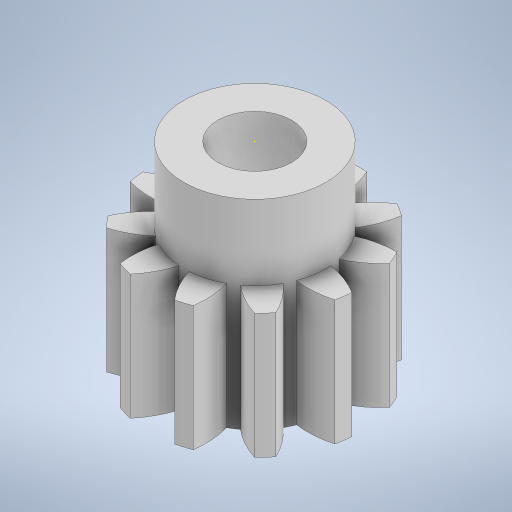
# Autodesk Inventor part: piniongear
Saved by Autodesk Inventor 2024 (Build 280153000, 153)
## iProperties
Created: 2024-05-02
Part Number: piniongear
Material: Generic
Document SubType Name: Modeling
Designer: maja6
Density: 1 g/cm^3
Appearance: Default
Author: maja6
Autodesk Inventor part; units mm, degrees
ref_plane "YZ Plane" through (0, 0, 0) normal (1, 0, 0) x (0, 1, 0)
ref_plane "XZ Plane" through (0, 0, 0) normal (0, 1, 0) x (-1, 0, 0)
ref_plane "XY Plane" through (0, 0, 0) normal (0, 0, 1) x (1, 0, 0)
sketch "Sketch1" plane through (0, 0, 0) normal (0, 0, 1) x (1, 0, 0)
  circle A0 centre (0, 0) radius 8.5
  dimension "d0" = 17
  constraints: 1 centre point, 1 coincident
  measures "d0" diameter of A0
extrude "Extrusion1" add sketch "Sketch1" along normal blind 5
spur gear teeth "Spur Gear1" teeth 11 pitch diameter 13.75 tip diameter 16.7792 root diameter 11.375 face width 5 trims to tip circle yes start plane through (0, 0, 5) normal (0, 0, 1) x (1, 0, 0)
sketch "Sketch2" plane through (0, 0, 5) normal (0, 0, 1) x (1, 0, 0)
  circle A0 centre (0, 0) radius 3.05
  circle A1 centre (0, 0) radius 5.6875
  point P0 (4.5531, 3.4084)
  dimension "d3" = 6.1
  constraints: 2 coincident, 1 centre point, 3 other
  measures "d3" diameter of A0
extrude "Extrusion2" add sketch "Sketch2" along normal blind 6
extrude "Extrusion3" cut sketch "Sketch2" against normal blind 6 contours A0
sketch "Sketch3" plane through (0, 0, 5) normal (0, 0, 1) x (1, 0, 0)
  line L0 (-1.9876, 4.927) -> (1.6861, 4.927)
  line L1 (1.6861, 4.927) -> (1.6861, 4.0217)
  line L2 (1.6861, 4.0217) -> (-1.9876, 4.0217)
  line L3 (-1.9876, 4.0217) -> (-1.9876, 4.927)
  point P0 (0, 0)
  constraints: 8 end point, 2 parallel, 1 horizontal, 1 perpendicular
sketch "Sketch4" plane through (0, 0, 11) normal (0, 0, 1) x (1, 0, 0)
  arc A0 (-1.209, 5.5575) -> (-1.9876, 5.3289) centre (0, 0) ccw projected
  line L0 (-1.9876, 5.3289) -> (1.9927, 5.3289)
  line L1 (1.9927, 5.3289) -> (1.9927, 4.1825)
  line L2 (1.9927, 4.1825) -> (-1.9876, 4.1825)
  line L3 (-1.9876, 4.1825) -> (-1.9876, 5.3289)
  constraints: 8 end point, 2 parallel, 1 horizontal, 1 perpendicular
extrude "Extrusion4" add sketch "Sketch4" along normal blind 6
sketch "Sketch5" plane through (-1.9876, 5.3289, 11) normal (0, 1, 0) x (1, 0, 0)
  circle A0 centre (1.9876, 3.0949) radius 1.5
  point P0 (1.9876, 11)
  dimension "d10" = 3
  constraints: 1 centre point
  measures "d10" diameter of A0
extrude "Extrusion5" cut sketch "Sketch5" along normal mid plane 30
sketch "Sketch6" plane through (-1.9876, 5.3289, 11) normal (0, 1, 0) x (1, 0, 0)
  line L0 (0, 0) -> (0, -6) projected
  line L1 (0, 0) -> (8.0095, 0)
  line L2 (8.0095, 0) -> (8.0095, -7.9416)
  line L3 (8.0095, -7.9416) -> (0, -7.9416)
  line L4 (0, -7.9416) -> (0, 0)
  point P0 (1.9876, 11)
  constraints: 8 end point, 2 parallel, 1 horizontal, 1 perpendicular
extrude "Extrusion6" cut sketch "Sketch6" against normal blind 30
thread "Thread1" size "M3x0.5" class "6H" standard "ANSI Metric M Profile" full length
thread "Thread2" size "M3x0.5" class "6H" standard "ANSI Metric M Profile" full length
sketch "Sketch7" plane through (0, 0, 11) normal (0, 0, 1) x (1, 0, 0)
  circle A0 centre (0, 0) radius 3.05
  circle A1 centre (0, 0) radius 2.95
  dimension "d19" = 5.9
  constraints: 2 centre point, 2 coincident
  measures "d19" diameter of A1
extrude "Extrusion7" add sketch "Sketch7" against normal blind 11
sketch "Sketch8" plane through (0, 0, 11) normal (0, 0, 1) x (1, 0, 0)
  circle A0 centre (0, 0) radius 2.95
  circle A1 centre (0, 0) radius 5.6875
  constraints: 2 centre point, 2 coincident
extrude "Extrusion8" add sketch "Sketch8" against normal blind 10
extrude "Extrusion9" add sketch "Sketch3" along normal blind 10
sketch "Sketch9" plane through (0, 0, 0) normal (0, 0, -1) x (-1, 0, 0)
  arc A0 (4.5531, 3.4084) -> (4.0217, 4.0217) centre (0, 0) ccw projected
  arc A1 (7.3634, 4.0207) -> (4.5531, 3.4084) centre (7.409, -2.9439) ccw projected
  arc A2 (7.8606, 2.9319) -> (7.3634, 4.0207) centre (0, 0) ccw projected
  arc A3 (5.5575, 1.209) -> (7.8606, 2.9319) centre (2.627, 7.5272) ccw projected
  arc A4 (5.673, 0.4057) -> (5.5575, 1.209) centre (0, 0) ccw projected
  arc A5 (8.3682, -0.5985) -> (5.673, 0.4057) centre (4.6413, -6.4821) ccw projected
  arc A6 (8.1979, -1.7833) -> (8.3682, -0.5985) centre (0, 0) ccw projected
  arc A7 (5.3289, -1.9876) -> (8.1979, -1.7833) centre (6.2795, 4.912) ccw projected
  arc A8 (4.9918, -2.7257) -> (5.3289, -1.9876) centre (0, 0) ccw projected
  arc A9 (6.7162, -5.0277) -> (4.9918, -2.7257) centre (0.4, -7.9624) ccw projected
  arc A10 (5.9324, -5.9324) -> (6.7162, -5.0277) centre (0, 0) ccw projected
  arc A11 (3.4084, -4.5531) -> (5.9324, -5.9324) centre (7.9383, 0.7373) ccw projected
  arc A12 (2.7257, -4.9918) -> (3.4084, -4.5531) centre (0, 0) ccw projected
  arc A13 (2.9319, -7.8606) -> (2.7257, -4.9918) centre (-3.9683, -6.9146) ccw projected
  arc A14 (1.7833, -8.1979) -> (2.9319, -7.8606) centre (0, 0) ccw projected
  arc A15 (0.4057, -5.673) -> (1.7833, -8.1979) centre (7.0767, -3.6715) ccw projected
  arc A16 (-0.4057, -5.673) -> (0.4057, -5.673) centre (0, 0) ccw projected
  arc A17 (-1.7833, -8.1979) -> (-0.4057, -5.673) centre (-7.0767, -3.6715) ccw projected
  arc A18 (-2.9319, -7.8606) -> (-1.7833, -8.1979) centre (0, 0) ccw projected
  arc A19 (-2.7257, -4.9918) -> (-2.9319, -7.8606) centre (3.9683, -6.9146) ccw projected
  arc A20 (-3.4084, -4.5531) -> (-2.7257, -4.9918) centre (0, 0) ccw projected
  arc A21 (-5.9324, -5.9324) -> (-3.4084, -4.5531) centre (-7.9383, 0.7373) ccw projected
  arc A22 (-6.7162, -5.0277) -> (-5.9324, -5.9324) centre (0, 0) ccw projected
  arc A23 (-4.9918, -2.7257) -> (-6.7162, -5.0277) centre (-0.4, -7.9624) ccw projected
  arc A24 (-5.3289, -1.9876) -> (-4.9918, -2.7257) centre (0, 0) ccw projected
  arc A25 (-8.1979, -1.7833) -> (-5.3289, -1.9876) centre (-6.2795, 4.912) ccw projected
  arc A26 (-8.3682, -0.5985) -> (-8.1979, -1.7833) centre (0, 0) ccw projected
  arc A27 (-5.673, 0.4057) -> (-8.3682, -0.5985) centre (-4.6413, -6.4821) ccw projected
  arc A28 (-5.5575, 1.209) -> (-5.673, 0.4057) centre (0, 0) ccw projected
  arc A29 (-7.8606, 2.9319) -> (-5.5575, 1.209) centre (-2.627, 7.5272) ccw projected
  arc A30 (-7.3634, 4.0207) -> (-7.8606, 2.9319) centre (0, 0) ccw projected
  arc A31 (-4.5531, 3.4084) -> (-7.3634, 4.0207) centre (-7.409, -2.9439) ccw projected
  arc A32 (-4.0217, 4.0217) -> (-4.5531, 3.4084) centre (0, 0) ccw projected
  arc A33 (-5.0277, 6.7162) -> (-4.0217, 4.0217) centre (1.8595, 7.7525) ccw projected
  arc A34 (-4.0207, 7.3634) -> (-5.0277, 6.7162) centre (0, 0) ccw projected
  arc A35 (-1.9876, 5.3289) -> (-4.0207, 7.3634) centre (-7.8244, 1.5291) ccw projected
  arc A36 (-1.209, 5.5575) -> (-1.9876, 5.3289) centre (0, 0) ccw projected
  arc A37 (-0.5985, 8.3682) -> (-1.209, 5.5575) centre (5.7556, 5.5165) ccw projected
  arc A38 (0.5985, 8.3682) -> (-0.5985, 8.3682) centre (0, 0) ccw projected
  arc A39 (1.209, 5.5575) -> (0.5985, 8.3682) centre (-5.7556, 5.5165) ccw projected
  arc A40 (1.9876, 5.3289) -> (1.209, 5.5575) centre (0, 0) ccw projected
  arc A41 (4.0207, 7.3634) -> (1.9876, 5.3289) centre (7.8244, 1.5291) ccw projected
  arc A42 (5.0277, 6.7162) -> (4.0207, 7.3634) centre (0, 0) ccw projected
  arc A43 (4.0217, 4.0217) -> (5.0277, 6.7162) centre (-1.8595, 7.7525) ccw projected
  circle A44 centre (0, 0) radius 2.95 projected
extrude "Extrusion10" add sketch "Sketch9" along normal blind 5
sketch "Sketch10" plane through (0, 0, 11) normal (0, 0, 1) x (1, 0, 0)
  point P0 (0, 0)
sketch "Sketch11" plane through (-1.9876, 4.0217, 11) normal (0, -1, 0) x (1, 0, 0)
  line L0 (3.6737, 4) -> (0, 4) projected
  line L1 (3.6737, 0) -> (3.6737, 4) projected
  line L2 (0, 4) -> (3.6737, 4)
  line L3 (3.6737, 4) -> (3.6737, 0)
  line L4 (3.6737, 0) -> (0, 0)
  line L5 (0, 0) -> (0, 4)
  point P0 (1.9876, -11)
  constraints: 8 end point, 2 parallel, 1 horizontal, 1 perpendicular
extrude "Extrusion11" cut sketch "Sketch11" against normal blind 10
body "Solid1"
